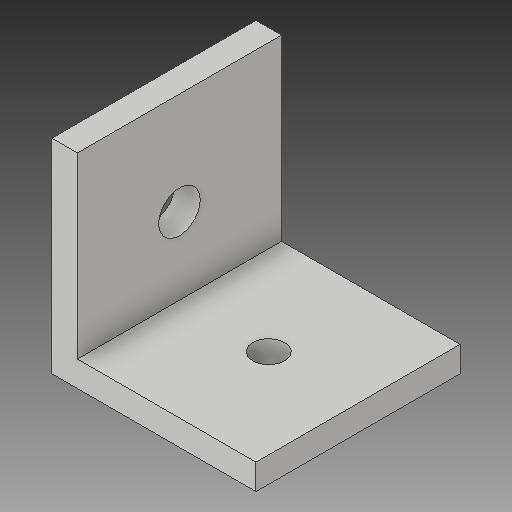
# Autodesk Inventor part: L-Bracket Bumper
Saved by Autodesk Inventor 2018 (Build 220112000, 112)
## iProperties
Created: 2019-01-20
Part Number: L-Bracket Bumper
Material: Generic
Document SubType Name: Modeling
Designer: maste
Density: 1 g/cm^3
Appearance: Default
Author: maste
Autodesk Inventor part; units mm, degrees
ref_plane "YZ Plane" through (0, 0, 0) normal (1, 0, 0) x (0, 1, 0)
ref_plane "XZ Plane" through (0, 0, 0) normal (0, 1, 0) x (-1, 0, 0)
ref_plane "XY Plane" through (0, 0, 0) normal (0, 0, 1) x (1, 0, 0)
sketch "Sketch1" plane through (0, 0, 0) normal (0, 0, 1) x (1, 0, 0)
  line L0 (0, 0) -> (3.175, 0)
  line L1 (3.175, 0) -> (3.175, 25.4)
  line L2 (3.175, 25.4) -> (0, 25.4)
  line L3 (0, 25.4) -> (0, 0)
  line L4 (0, 0) -> (25.4, 0)
  line L5 (25.4, 0) -> (25.4, 3.175)
  line L6 (25.4, 3.175) -> (0, 3.175)
  line L7 (0, 3.175) -> (0, 0)
  dimension "d0" = 3.175
  dimension "d1" = 25.4
  dimension "d2" = 25.4
  dimension "d3" = 3.175
  constraints: 16 end point, 4 parallel, 2 horizontal, 2 perpendicular
  measures "d0" distance of L2.end L1.end
  measures "d1" distance of L1.end L0.end
  measures "d2" distance of L6.end L5.end
  measures "d3" distance of L5.end L4.end
extrude "Extrusion1" add sketch "Sketch1" along normal blind 25.4
sketch "Sketch2" plane through (3.175, 3.175, 0) normal (0, 1, 0) x (1, 0, 0)
  line L0 (22.225, 0) -> (0, 0) construction
  line L1 (11.1125, 0) -> (11.1125, -12.7) construction
  line L2 (11.1125, 0) -> (23.8125, 0) construction
  circle A0 centre (11.1125, -12.7) radius 1.9812
  point P0 (-3.175, 0)
  dimension "d6" = 12.7
  dimension "d7" = 90
  dimension "d8" = 3.9624
  constraints: 4 end point, 1 centre point, 1 coincident, 1 horizontal, 1 midpoint, 1 perpendicular, 1 vertical
  measures "d6" distance of L1.start L1.end
  measures "d7" angle of L1 L2
  measures "d8" diameter of A0
extrude "Extrusion2" cut sketch "Sketch2" against normal blind 25.4
sketch "Sketch3" plane through (3.175, 3.175, 0) normal (1, 0, 0) x (0, 0, -1)
  line L0 (0, 22.225) -> (-25.4, 22.225) construction
  circle A0 centre (-12.7, 9.525) radius 2.5797
  line L1 (-12.7, 9.525) -> (-12.7, 22.225)
  point P0 (0, -3.175)
  dimension "d11" = 5.1594
  dimension "d14" = 12.7
  constraints: 2 end point, 1 centre point, 1 midpoint
  measures "d11" diameter of A0
  measures "d14" distance of L1.start L1.end
extrude "Extrusion3" cut sketch "Sketch3" against normal blind 25.4
body "Solid1"
